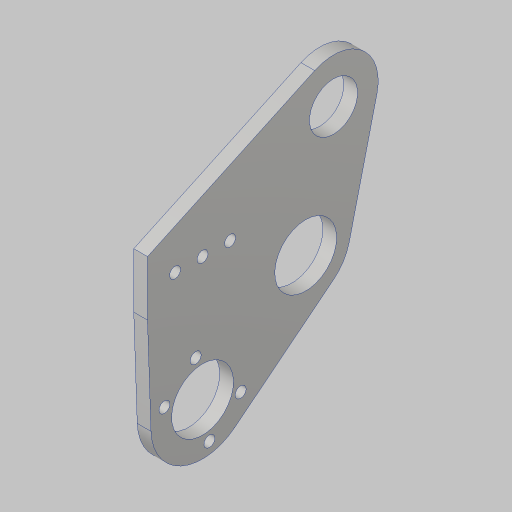
# Autodesk Inventor part: GP5-011
Saved by Autodesk Inventor 2023.5 (Build 275446000, 446)
## iProperties
Created: 2025-02-03
Part Number: GP5-011
Material: Aluminum 6061
Document SubType Name: Modeling
Designer: slick
Density: 2.7 g/cm^3
Appearance: Aluminum - Flat
Author: slick
Autodesk Inventor part; units mm, degrees
ref_plane "YZ Plane" through (0, 0, 0) normal (1, 0, 0) x (0, 1, 0)
ref_plane "XZ Plane" through (0, 0, 0) normal (0, 1, 0) x (-1, 0, 0)
ref_plane "XY Plane" through (0, 0, 0) normal (0, 0, 1) x (1, 0, 0)
sketch "Sketch1" plane through (0, 0, 0) normal (1, 0, 0) x (0, 1, 0)
  line L0 (-12.7, 25.4) -> (12.7, 25.4) construction
  line L1 (12.7, 25.4) -> (12.7, -25.4) construction
  line L2 (12.7, -25.4) -> (-12.7, -25.4) construction
  line L3 (-12.7, -25.4) -> (-12.7, 25.4) construction
  line L4 (-12.7, 25.4) -> (12.7, -25.4) construction
  line L5 (12.7, 25.4) -> (-12.7, -25.4) construction
  circle A0 centre (-57.15, 0) radius 14.2875
  circle A1 centre (-127, -49.5046) radius 38.1 construction
  circle A2 centre (-57.15, 0) radius 23.8125 construction
  circle A3 centre (66.2076, -50.8) radius 5.9531 construction
  circle A4 centre (29.7638, -60.4629) radius 31.75 construction
  circle A5 centre (66.2076, -50.8) radius 17.4625 construction
  circle A6 centre (66.2076, -50.8) radius 22.098 construction
  line L6 (12.7, -25.4) -> (215.9, -25.4) construction
  line L7 (215.9, -25.4) -> (215.9, 25.4) construction
  line L8 (215.9, 25.4) -> (12.7, 25.4) construction
  line L9 (-57.9919, 23.7976) -> (-12.7, 25.4)
  line L10 (-12.7, 25.4) -> (12.7, 25.4)
  line L11 (12.7, 25.4) -> (48.4866, -51.7818)
  arc A7 (-57.9919, 23.7976) -> (-75.7842, -14.8258) centre (-57.15, 0) ccw
  circle A8 centre (29.7638, -60.4629) radius 12.7 construction
  circle A9 centre (-23.3158, -47.625) radius 41.91 construction
  circle A10 centre (-23.3158, -47.625) radius 20.32 construction
  circle A11 centre (-57.15, 0) radius 38.1 construction
  circle A12 centre (29.7638, -60.4629) radius 11.1125
  circle A13 centre (-23.3158, -47.625) radius 14.2875
  circle A14 centre (29.7638, -60.4629) radius 20.6375 construction
  circle A15 centre (-23.3158, -47.625) radius 20.6375 construction
  line L12 (24.9123, -80.5221) -> (-28.1673, -67.6841)
  line L13 (-39.4654, -60.474) -> (-75.7842, -14.8258)
  arc A16 (24.9123, -80.5221) -> (48.4866, -51.7818) centre (29.7638, -60.4629) ccw
  arc A17 (-39.4654, -60.474) -> (-28.1673, -67.6841) centre (-23.3158, -47.625) ccw
  circle A18 centre (40.8076, -31.75) radius 6.35 construction
  line L14 (-62.9316, -17.5873) -> (-75.389, -3.175) construction
  line L15 (-75.389, -3.175) -> (-51.3684, 17.5873) construction
  line L16 (-51.3684, 17.5873) -> (-38.911, 3.175) construction
  line L17 (-38.911, 3.175) -> (-62.9316, -17.5873) construction
  line L18 (-62.9316, -17.5873) -> (-51.3684, 17.5873) construction
  line L19 (-75.389, -3.175) -> (-38.911, 3.175) construction
  point P0 (0, 0)
  point P1 (0, -12.7)
  point P2 (0, 0)
  point P3 (0, 12.7)
  point P4 (77.6113, -69.7282)
  point P5 (-39.5444, 23.7687)
  point P6 (74.3671, -50.8)
  point P7 (66.2076, -68.2625)
  point P8 (85.4103, -66.5975)
  point P9 (93.5697, -49.135)
  point P10 (82.5265, -33.3375)
  point P11 (63.3238, -35.0025)
  point P12 (55.1644, -52.465)
  dimension "d20" = 34.925
  dimension "d21" = 44.196
  dimension "d0" = 25.4
  dimension "d1" = 50.8
  dimension "d2" = 28.575
  dimension "d3" = 57.15
  dimension "d4" = 76.2
  dimension "d5" = 127
  dimension "d6" = 49.5046
  dimension "d11" = 12.7
  dimension "d12" = 12.7
  dimension "d13" = 9.525
  dimension "d18" = 11.9062
  dimension "d19" = 63.5
  dimension "d22" = 203.2
  dimension "d23" = 25.4
  dimension "d24" = 53.5076
  dimension "d31" = 360
  dimension "d40" = 25.4
  dimension "d41" = 83.82
  dimension "d42" = 40.64
  dimension "d43" = 76.2
  dimension "d44" = 36.4438
  dimension "d46" = 6.35
  dimension "d48" = 12.7
  dimension "d49" = 25.4
  dimension "d50" = 22.225
  dimension "d51" = 31.75
  dimension "d52" = 19.05
  dimension "d54" = 3.175
  dimension "d62" = 22.225
  constraints: 40 end point, 17 centre point, 16 coincident, 12 point on circle, 10 tangent, 5 vertical alignment, 4 parallel, 4 perpendicular, 3 equal radius, 3 midpoint, 2 horizontal, 1 horizontal alignment, 12 other
  measures "d0" distance of L1.end L2.end
  measures "d1" distance of L0.end L1.end
  measures "d2" diameter of A0
  measures "d3" distance of A0.centre point (0, 0)
  measures "d4" diameter of A1
  measures "d5" horizontal distance of A1.centre point (0, 0)
  measures "d6" vertical distance of A1.centre point (0, 0)
  measures "d11" distance of point (0, -12.7) point (0, 0)
  measures "d12" distance of point (0, 0) point (0, 12.7)
  measures "d13" radial gap between concentric circles of A0 A2
  measures "d18" diameter of A3
  measures "d19" diameter of A4
  measures "d22" distance between parallel lines of L1 L7
  measures "d23" distance from line of L6 point (66.208, -50.8)
  measures "d24" horizontal distance of L1.end A3.centre
  measures "d40" diameter of A8
  measures "d41" diameter of A9
  measures "d42" diameter of A10
  measures "d43" diameter of A11
  measures "d44" horizontal distance of A3.centre A4.centre
  measures "d46" radial gap between concentric circles of A13 A15
  measures "d48" diameter of A18
  measures "d49" horizontal distance of A18.centre A3.centre
  measures "d50" diameter of A12
  measures "d51" distance of L14.end L15.end
  measures "d52" distance of L14.end L14.start
  measures "d54" vertical distance of L16.end point (0, 0)
  measures "d62" vertical distance of L2.end A10.centre
extrude "Extrusion1" add sketch "Sketch1" along normal blind 6.35
hole "Hole1" at (0, 0, -12.7) at (0, 0, 0) at (0, 0, 12.7) direction (1, 0, 0) diameter 5.1054 end through all clearance for "Flat Head Machine Screw (82)" size "#10" standard "Ansi Unified Screw Threads"
hole "Hole2" at (0, -75.389, -3.175) at (0, -62.9316, -17.5873) at (0, -38.911, 3.175) at (0, -51.3684, 17.5873) direction (1, 0, 0) diameter 5.1054 end through all clearance for "Flat Head Machine Screw (82)" size "#10" standard "Ansi Unified Screw Threads"
equation "\"d12\" = d11"
body "Solid1"
